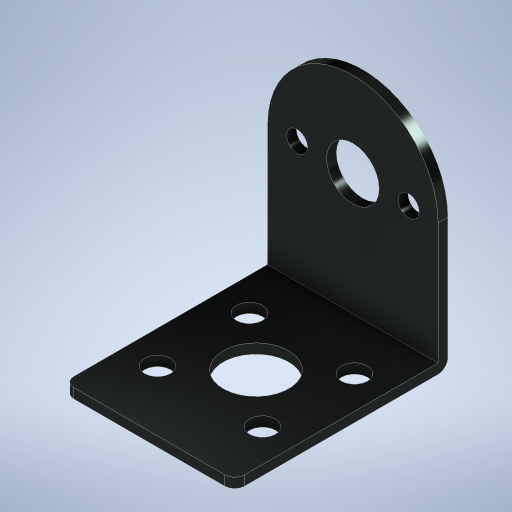
# Autodesk Inventor part: WH-Bracket-JGA25A
Saved by Autodesk Inventor 2024.2 (Build 282272000, 272)
## iProperties
Created: 2025-06-30
Part Number: WH-Bracket-JGA25A
Material: Generic
Document SubType Name: Modeling
Designer: Admin
Density: 1 g/cm^3
Appearance: Gunmetal - Polished
Author: Admin
Autodesk Inventor part; units mm, degrees
ref_plane "YZ Plane" through (0, 0, 0) normal (1, 0, 0) x (0, 1, 0)
ref_plane "XZ Plane" through (0, 0, 0) normal (0, 1, 0) x (-1, 0, 0)
ref_plane "XY Plane" through (0, 0, 0) normal (0, 0, 1) x (1, 0, 0)
sketch "Sketch1" plane through (0, 0, 0) normal (0, 0, 1) x (1, 0, 0)
  arc A0 (13, 0) -> (-13, 0) centre (0, 0) ccw
  circle A1 centre (0, 0) radius 4
  line L0 (0, 13) -> (0, -20) construction
  line L1 (-13, 0) -> (-13, -20)
  line L2 (-13, -20) -> (13, -20)
  line L3 (13, -20) -> (13, 0)
  circle A2 centre (8.5, 0) radius 1.6
  circle A3 centre (-8.5, 0) radius 1.6
  line L4 (-13, -18.5) -> (13, -18.5)
  dimension "d1" = 13
  dimension "d2" = 33
  dimension "d3" = 3.2
  dimension "d4" = 8.5
  dimension "d5" = 8
  dimension "d6" = 1.5
  constraints: 10 end point, 4 centre point, 3 perpendicular, 3 point on circle, 2 coincident, 2 point on line, 2 vertical, 1 symmetric about line, 1 tangent, 1 other
  measures "d1" radius of A0
  measures "d2" distance of L0.start L0.end
  measures "d3" diameter of A2
  measures "d4" distance of A2.centre point (0, 0)
  measures "d5" diameter of A1
  measures "d6" distance between parallel lines of L2 L4
extrude "Extrusion1" add sketch "Sketch1" along normal blind 1.5 contours L3 L4 L1 A0
extrude "Extrusion2" add sketch "Sketch1" along normal blind 32.5 contours L3 L2 L1 L4
fillet "Fillet1" radius 1.5 3 edges at (-13, -19.25, 32.5) (13, -19.25, 32.5) (0, -20, 0)
sketch "Sketch2" plane through (-13, -20, 1.5) normal (0, -1, 0) x (1, 0, 0)
  arc A0 (26, 29.5) -> (24.5, 31) centre (24.5, 29.5) ccw projected
  line L0 (26, 0) -> (0, 0) projected
  line L1 (26, 29.5) -> (0, 0) construction
  line L2 (0, 0) -> (0, 29.5) projected
  line L3 (26, 0) -> (0, 29.5) construction
  line L4 (13, 14.75) -> (13, 0) construction
  circle A1 centre (21, 7.75) radius 2
  circle A2 centre (13, 14.75) radius 5
  circle A3 centre (5, 7.75) radius 2
  line L5 (13, 14.75) -> (0, 14.75) construction
  circle A4 centre (21, 21.75) radius 2
  circle A5 centre (5, 21.75) radius 2
  point P0 (13, -1.5)
  dimension "d13" = 4
  dimension "d14" = 8
  dimension "d15" = 7
  dimension "d16" = 10
  constraints: 8 end point, 5 centre point, 4 midpoint, 3 symmetric about line, 1 coincident, 3 other
  measures "d13" diameter of A1
  measures "d14" distance from line of A1.centre L4
  measures "d15" vertical distance of point (13, 14.75) A1.centre
  measures "d16" diameter of A2
extrude "Extrusion3" cut sketch "Sketch2" against normal through all
body "Solid1"
